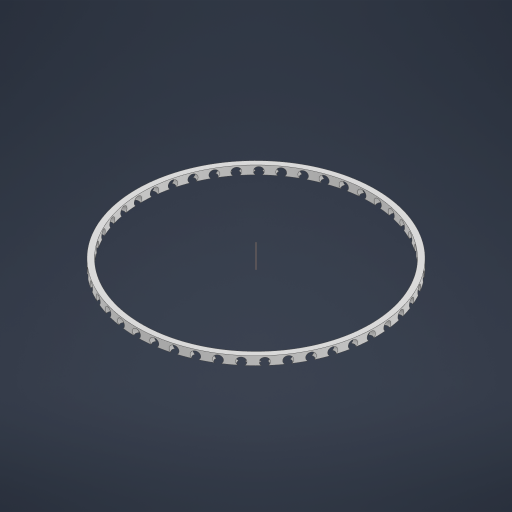
# Autodesk Inventor part: Large Bearing Spacer
Saved by Autodesk Inventor 2023 (Build 270158000, 158)
## iProperties
Created: 2022-11-20
Part Number: Large Bearing Spacer
Material: Generic
Document SubType Name: Modeling
Designer: Izack Waczko
Density: 1 g/cm^3
Appearance: Default
Author: Izack Waczko
Autodesk Inventor part; units mm, degrees
ref_plane "YZ Plane" through (0, 0, 0) normal (1, 0, 0) x (0, 1, 0)
ref_plane "XZ Plane" through (0, 0, 0) normal (0, 1, 0) x (-1, 0, 0)
sketch "Sketch1" plane through (0, 0, 0) normal (0, 1, 0) x (-1, 0, 0)
  circle A0 centre (0, 0) radius 54.867 construction
  circle A1 centre (0, 0) radius 53.617
  circle A2 centre (0, 0) radius 56.117
  dimension "d0" = 109.734
  dimension "d1" = 2.5
  dimension "d3" = 1.25
  constraints: 3 centre point, 3 coincident
  measures "d0" diameter of A0
  measures "d1" radial gap between concentric circles of A2 A1
  measures "d3" radial gap between concentric circles of A1 A0
extrude "Extrusion1" add sketch "Sketch1" along normal blind 4
ref_plane "Work Plane1" through (0, 1.5, 0) normal (0, 1, 0) x (1, 0, 0)
sketch "Sketch2" plane through (0, 1.5, 0) normal (0, 1, 0) x (1, 0, 0)
  circle A0 centre (0, 0) radius 56.117 projected
  circle A1 centre (0, 0) radius 53.617 projected
  circle A2 centre (0, 0) radius 56.117 construction
  line L0 (0, -56.117) -> (0, -53.617) construction
  circle A3 centre (0, 0) radius 53.617 construction
  circle A4 centre (0, -54.867) radius 2.25
  line L1 (0, -57.117) -> (0, -52.617)
  dimension "d7" = 4.5
  constraints: 4 end point, 2 point on circle, 2 vertical alignment, 1 centre point, 1 midpoint, 1 point on line, 1 vertical, 2 other
  measures "d7" diameter of A4
revolve "Revolution1" cut sketch "Sketch2" angle 360 about axis through (0, 1.5, 57.117) along (0, 0, -1) picked at (-1.5776, -54.933) picked at (-0.3956, -56.4259) picked at (-0.3846, -53.3042) contours A4 A1 L1 A0 | A0 L1 A4 | A4 L1 A1
pattern_circular "Circular Pattern1" count 45 over 360 about axis through (0, 0, 0) along (0, 1, 0) of "Revolution1"
body "Solid1"
